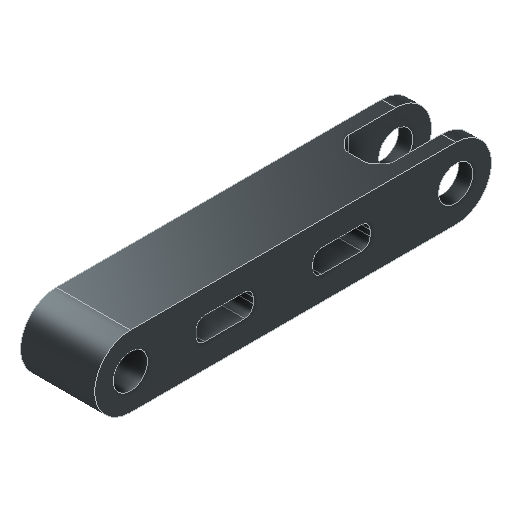
# Autodesk Inventor part: Link_OC
Saved by Autodesk Inventor 2026.2 (Build 302298000, 298)
## iProperties
Created: 2025-12-26
Part Number: Link_OC
Material: ABS 塑膠
Document SubType Name: Modeling
Designer: Hsiangyu
Mass: 54.6026 g
Surface Area: 155.33 cm^2
Volume: 54.6026 cm^3
Density: 1.06 g/cm^3
Appearance: 鐵灰色
Author: Hsiangyu
Autodesk Inventor part; units mm, degrees
ref_plane "YZ Plane" through (0, 0, 0) normal (1, 0, 0) x (0, 1, 0)
ref_plane "XZ Plane" through (0, 0, 0) normal (0, 1, 0) x (-1, 0, 0)
ref_plane "XY Plane" through (0, 0, 0) normal (0, 0, 1) x (1, 0, 0)
sketch "草圖1" plane through (0, 0, 0) normal (1, 0, 0) x (0, 1, 0)
  line L0 (0, 0) -> (0, -113.9)
  circle A0 centre (0, 0) radius 6
  circle A1 centre (0, -113.9) radius 6
  circle A2 centre (0, 0) radius 12.5
  circle A3 centre (0, -113.9) radius 12.5
  line L1 (12.5, 0) -> (12.5, -113.9)
  line L2 (-12.5, 0) -> (-12.5, -113.9)
  line L3 (4, -23) -> (-4, -23)
  line L4 (-4, -23) -> (-4, -43)
  line L5 (-4, -43) -> (4, -43)
  line L6 (4, -43) -> (4, -23)
  line L7 (4, -63.9) -> (-4, -63.9)
  line L8 (-4, -63.9) -> (-4, -83.9)
  line L9 (-4, -83.9) -> (4, -83.9)
  line L10 (4, -83.9) -> (4, -63.9)
  line L11 (12.5, -92) -> (-12.5, -92)
  point P0 (0, -23)
  point P1 (0, -63.9)
  dimension "d0" = 113.9
  dimension "d1" = 12
  dimension "d2" = 25
  dimension "d5" = 20
  dimension "d7" = 8
  dimension "d8" = 23
  dimension "d9" = 30
  dimension "d11" = 92
  constraints: 24 end point, 4 centre point, 4 coincident, 4 parallel, 4 point on circle, 4 tangent, 3 perpendicular, 2 equal length, 2 equal radius, 2 horizontal, 2 midpoint, 2 point on line, 2 vertical alignment, 1 vertical
  measures "d0" distance of L0.start L0.end
  measures "d1" diameter of A0
  measures "d2" diameter of A2
  measures "d5" distance of L5.end L3.start
  measures "d7" distance of L3.start L3.end
  measures "d8" distance from line of L0.start L3
  measures "d9" distance from line of L0.end L9
  measures "d11" distance from line of L0.start L11
extrude "擠出1" add sketch "草圖1" along normal mid plane 16 contours A2 L1 L11 L0 L9 L10 L7 L5 L6 L3 | L0 L3 L4 L5 L7 L8 L9 L11 L2 A2 | A2
sketch "草圖4" plane through (8, 0, 0) normal (1, 0, 0) x (0, 0, -1)
  line L0 (63.9, -4) -> (63.9, 4) projected
  line L1 (63.9, 4) -> (83.9, 4) projected
  line L2 (83.9, 4) -> (83.9, -4) projected
  line L3 (83.9, -4) -> (63.9, -4) projected
  line L4 (43, 4) -> (43, -4) projected
  line L5 (43, -4) -> (23, -4) projected
  line L6 (23, -4) -> (23, 4) projected
  line L7 (23, 4) -> (43, 4) projected
  circle A0 centre (0, 0) radius 6 projected
  line L8 (92, 12.5) -> (0, 12.5) projected
  arc A1 (0, 12.5) -> (0, -12.5) centre (0, 0) ccw projected
  line L9 (0, -12.5) -> (92, -12.5) projected
  line L10 (0, 12.5) -> (113.9, 12.5) projected
  line L11 (0, -12.5) -> (113.9, -12.5) projected
  circle A2 centre (113.9, 0) radius 12.5 projected
  circle A3 centre (113.9, 0) radius 6 projected
  point P0 (96, -12.5)
  point P1 (96, 12.5)
extrude "擠出4" add sketch "草圖4" along normal blind 5
sketch "草圖5" plane through (-8, 0, 0) normal (-1, 0, 0) x (0, 0, 1)
  line L0 (-92, -12.5) -> (0, -12.5) projected
  arc A0 (0, -12.5) -> (0, 12.5) centre (0, 0) ccw projected
  line L1 (0, 12.5) -> (-92, 12.5) projected
  circle A1 centre (0, 0) radius 6 projected
  line L2 (-43, -4) -> (-43, 4) projected
  line L3 (-43, 4) -> (-23, 4) projected
  line L4 (-23, 4) -> (-23, -4) projected
  line L5 (-23, -4) -> (-43, -4) projected
  line L6 (-63.9, 4) -> (-63.9, -4) projected
  line L7 (-63.9, -4) -> (-83.9, -4) projected
  line L8 (-83.9, -4) -> (-83.9, 4) projected
  line L9 (-83.9, 4) -> (-63.9, 4) projected
  line L10 (0, -12.5) -> (-113.9, -12.5) projected
  line L11 (0, 12.5) -> (-113.9, 12.5) projected
  circle A2 centre (-113.9, 0) radius 12.5 projected
  circle A3 centre (-113.9, 0) radius 6 projected
extrude "擠出5" add sketch "草圖5" along normal blind 5
chamfer "倒角2" distance 4 angle 45 2 edges at (-8, 0, -92) (8, 0, -92)
fillet "圓角4" radius 3 4 edges at (-8, 0, -96) (-4, 0, -92) (4, 0, -92) (8, 0, -96)
fillet "圓角5" radius 3 8 edges at (0, 4, -23) (0, -4, -23) (0, -4, -43) (0, 4, -43) (0, 4, -63.9) (0, -4, -63.9) (0, -4, -83.9) (0, 4, -83.9)
